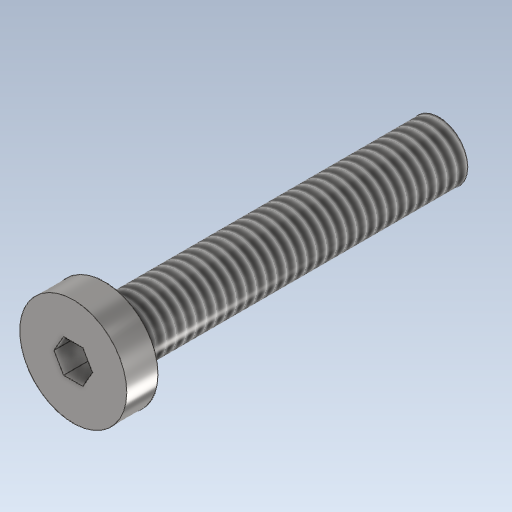
# Autodesk Inventor part: M2_6-15
Saved by Autodesk Inventor 2020.4 (Build 244396000, 396)
## iProperties
Created: 2021-09-11
Part Number: M2_6-15
Material: チタン
Document SubType Name: Modeling
Designer: Masato Kubotera
Density: 6.42573 g/cm^3
Appearance: 半つや出し
Mass: 0.657 g
Surface Area: 1.87099 cm^2
Volume: 0.102245 cm^3
Description: ネジ
Author: Masato Kubotera
Autodesk Inventor part; units mm, degrees
ref_plane "YZ Plane" through (0, 0, 0) normal (1, 0, 0) x (0, 1, 0)
ref_plane "XZ Plane" through (0, 0, 0) normal (0, 1, 0) x (-1, 0, 0)
ref_plane "XY Plane" through (0, 0, 0) normal (0, 0, 1) x (1, 0, 0)
sketch "スケッチ1" plane through (0, 0, 0) normal (1, 0, 0) x (0, 1, 0)
  line L0 (0, 16.4) -> (0, 0)
  line L1 (0, 0) -> (2.4, 0)
  line L2 (2.4, 0) -> (2.4, 1.4)
  line L3 (2.4, 1.4) -> (1.3, 1.4)
  line L4 (1.3, 1.4) -> (1.3, 16.4)
  line L5 (1.3, 16.4) -> (0, 16.4)
  dimension "d1" = 1.3
  dimension "d2" = 1.4
  dimension "d3" = 2.4
  dimension "d10" = 15
  constraints: 12 end point, 5 perpendicular, 1 vertical
  measures "d1" distance of L0.start L4.end
  measures "d2" distance of L1.end L2.end
  measures "d3" distance of L1.end L0.end
  measures "d10" distance of L3.end L4.end
revolve "回転1" add sketch "スケッチ1" angle 360 about axis through (0, 0, 16.4) along (0, 0, -1)
thread "ねじ1" size "M2.6x0.45" class "6g" standard "ANSI Metric M Profile" full length
sketch "スケッチ2" plane through (0, 0, 0) normal (0, 0, -1) x (-1, 0, 0)
  line L0 (0, 0.866) -> (0.75, 0.433)
  line L1 (0.75, 0.433) -> (0.75, -0.433)
  line L2 (0.75, -0.433) -> (0, -0.866)
  line L3 (0, -0.866) -> (-0.75, -0.433)
  line L4 (-0.75, -0.433) -> (-0.75, 0.433)
  line L5 (-0.75, 0.433) -> (0, 0.866)
  line L6 (0, 2.4) -> (0, -2.4) construction
  circle A0 centre (0, 0) radius 2.4 projected
  point P0 (0, 0)
  point P1 (0, 0)
  dimension "d7" = 1.5
  constraints: 14 end point, 2 point on circle, 1 coincident, 1 midpoint, 1 point on line, 1 vertical, 13 other
  measures "d7" distance between parallel lines of L1 L4
extrude "押し出し1" cut sketch "スケッチ2" against normal blind 1.4 contours L0 L1 L2 L3 L4 L5
